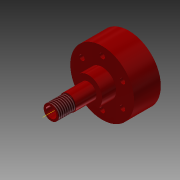
# Autodesk Inventor part: wheel_hub_spacer
Saved by Autodesk Inventor 2014 (Build 180170000, 170)
## iProperties
Created: 2014-03-12
Part Number: wheel_hub_spacer
Material: Aluminium 6061
Document SubType Name: Modeling
Designer: Yann
Density: 2.71 g/cm^3
Appearance: Rouge
Mass: 202.518 g
Surface Area: 172.85 cm^2
Volume: 74.7298 cm^3
d0: 30,000 mm
d1: 13,000 mm
d2: 7,500 mm
d5: 13,000 mm
d6: 25,000 mm
d8: 10,000 mm
d10: 0,00 deg
d11: 5,000 mm
d12: 22,000 mm
d14: 0,00 deg
d15: 6,000 nd
d16: 360,00 deg
d23: 7,000 mm
d25: 19,000 mm
d26: 16,000 mm
Author: Yann
Autodesk Inventor part; units mm, degrees
ref_plane "YZ Plane" through (0, 0, 0) normal (1, 0, 0) x (0, 1, 0)
ref_plane "XZ Plane" through (0, 0, 0) normal (0, 1, 0) x (-1, 0, 0)
ref_plane "XY Plane" through (0, 0, 0) normal (0, 0, 1) x (1, 0, 0)
sketch "esq_rev" plane through (0, 0, 0) normal (0, 0, 1) x (1, 0, 0)
  line L0 (0, -40.1) -> (0, 62.1) projected
  line L1 (7.5, -9.5) -> (7.5, 9.5)
  line L2 (7.5, 9.5) -> (13, 9.5)
  line L3 (13, 9.5) -> (13, 22.5)
  line L4 (13, 22.5) -> (30, 22.5)
  line L5 (30, 22.5) -> (30, 47.5)
  line L6 (30, 47.5) -> (0, 47.5)
  line L7 (0, -25.5) -> (0, -0.0006)
  line L8 (-38.091, 0) -> (41.3485, 0) projected
  line L9 (-26.7425, 30) -> (-5.3911, 30) projected
  line L10 (-5.3911, 30) -> (28.4337, 30) projected
  line L11 (28.4337, 30) -> (7.0823, 30) projected
  line L12 (7.0823, 30) -> (-26.7425, 30) projected
  line L13 (-6.854, 30) -> (-23.5883, 30) projected
  line L14 (-23.5883, 30) -> (-14.3845, 30) projected
  line L15 (-4.5388, 30) -> (-6.854, 30) projected
  line L16 (-24.4454, 30) -> (5.2291, 30) projected
  line L17 (5.2291, 30) -> (2.6006, 30) projected
  line L18 (-13.9964, 30) -> (-24.4454, 30) projected
  line L19 (24.4454, 30) -> (-5.2291, 30) projected
  line L20 (-5.2291, 30) -> (-2.6006, 30) projected
  line L21 (13.9964, 30) -> (24.4454, 30) projected
  line L22 (4.5388, 30) -> (7.194, 30) projected
  line L23 (7.194, 30) -> (24.9396, 30) projected
  line L24 (24.9396, 30) -> (14.3845, 30) projected
  line L25 (-4.5388, 30) -> (-14.5, 30) projected
  line L26 (2.6006, 30) -> (-13.9964, 30) projected
  line L27 (13.9964, 30) -> (-2.6006, 30) projected
  line L28 (14.5, 30) -> (4.5388, 30) projected
  line L29 (-12.5, 30) -> (12.5, 30) projected
  line L30 (-12.5, -20) -> (12.5, -20) projected
  line L31 (7, -9.5) -> (7, -25.5)
  line L32 (7, -25.5) -> (0, -25.5)
  line L33 (7, -9.5) -> (7.5, -9.5)
  line L34 (0, -0.0006) -> (0, 47.5)
  point P0 (0, 0)
  dimension "d0" = 30
  dimension "d1" = 13
  dimension "d2" = 7.5
  dimension "d5" = 13
  dimension "d6" = 25
  dimension "d23" = 7
  dimension "d25" = 19
  dimension "d26" = 16
  constraints: 22 end point, 3 horizontal, 2 collinear, 2 perpendicular, 2 vertical, 1 parallel, 1 point on line, 1 other
  measures "d0" distance between parallel lines of L0 L5
  measures "d1" distance between parallel lines of L0 L3
  measures "d2" distance between parallel lines of L1 L0
  measures "d5" distance of L2.end L3.end
  measures "d6" distance of L4.end L5.end
  measures "d23" distance between parallel lines of L0 L31
  measures "d25" distance between parallel lines of L33 L2
  measures "d26" distance between parallel lines of L33 L32
revolve "rev" add sketch "esq_rev" angle 360 about axis through (0, -25.5, 0) along (0, 1, 0)
sketch "esq_percage" plane through (0, 0, 0) normal (0, 1, 0) x (-1, 0, 0)
  line L0 (0, -7) -> (0, 7) projected
  line L1 (-7, 0) -> (7, 0) projected
  circle A0 centre (0, 0) radius 5
  dimension "d8" = 10
  constraints: 1 centre point, 1 coincident
  measures "d8" diameter of A0
extrude "ext_percage" cut sketch "esq_percage" along normal through all both and the other way through all
sketch "Esq_trous" plane through (0, 0, 0) normal (0, 1, 0) x (-1, 0, 0)
  line L0 (0, -4.9) -> (0, 29.4) projected
  line L1 (-3.5, 0) -> (3.5, 0) projected
  circle A0 centre (0, 22) radius 2.5
  point P0 (0, 0)
  dimension "d11" = 5
  dimension "d12" = 22
  constraints: 1 centre point, 1 point on line
  measures "d11" diameter of A0
  measures "d12" distance of A0.centre point (0, 0)
extrude "ext_trous" cut sketch "Esq_trous" along normal through all
pattern_circular "Réseau circulaire1" count 6 over 360 about axis through (0, -10, 0) along (0, 1, 0) of "ext_trous"
thread "Filetage2" size "M14x2" class "6g" standard "ANSI Metric M Profile" full length
